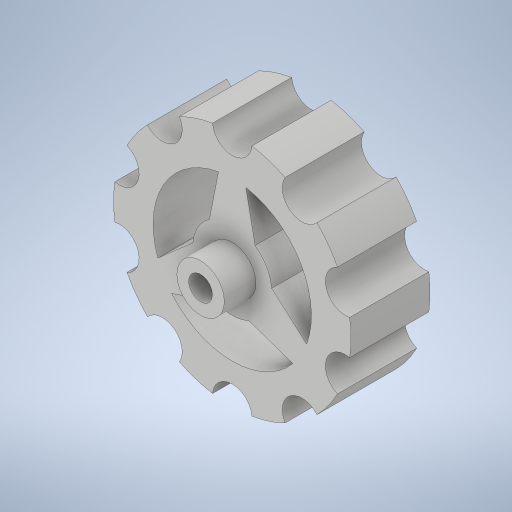
# Autodesk Inventor part: Guntas_Wheel_New
Saved by Autodesk Inventor 2024 (Build 280153000, 153)
## iProperties
Created: 2023-06-29
Part Number: Guntas_Wheel_New
Material: Generic
Document SubType Name: Modeling
Designer: gaura
Density: 1 g/cm^3
Appearance: Default
Author: gaura
Autodesk Inventor part; units mm, degrees
ref_plane "YZ Plane" through (0, 0, 0) normal (1, 0, 0) x (0, 1, 0)
ref_plane "XZ Plane" through (0, 0, 0) normal (0, 1, 0) x (-1, 0, 0)
ref_plane "XY Plane" through (0, 0, 0) normal (0, 0, 1) x (1, 0, 0)
sketch "Sketch1" plane through (0, 0, 0) normal (0, 0, 1) x (1, 0, 0)
  circle A0 centre (0, 0) radius 75
  dimension "d0" = 150
  constraints: 1 centre point, 1 coincident
  measures "d0" diameter of A0
extrude "Extrusion1" add sketch "Sketch1" along normal mid plane 50
sketch "Sketch2" plane through (0, 0, 0) normal (0, 0, 1) x (1, 0, 0)
  circle A0 centre (0, 0) radius 50
  dimension "d3" = 100
  constraints: 1 centre point, 1 coincident
  measures "d3" diameter of A0
extrude "Extrusion2" cut sketch "Sketch2" along normal mid plane 50
sketch "Sketch3" plane through (0, 0, 0) normal (0, 0, 1) x (1, 0, 0)
  circle A0 centre (0, 0) radius 25
  dimension "d6" = 50
  constraints: 1 centre point, 1 coincident
  measures "d6" diameter of A0
extrude "Extrusion3" add sketch "Sketch3" along normal mid plane 50
sketch "Sketch10" plane through (0, 0, 25) normal (0, 0, 1) x (1, 0, 0)
  circle A0 centre (0, 0) radius 75 projected
  circle A1 centre (0, 75) radius 12.5
  circle A2 centre (-44.0839, 60.6763) radius 12.5
  circle A3 centre (-71.3292, 23.1763) radius 12.5
  circle A4 centre (-71.3292, -23.1763) radius 12.5
  circle A5 centre (-44.0839, -60.6763) radius 12.5
  circle A6 centre (0, -75) radius 12.5
  circle A7 centre (44.0839, -60.6763) radius 12.5
  circle A8 centre (71.3292, -23.1763) radius 12.5
  circle A9 centre (71.3292, 23.1763) radius 12.5
  circle A10 centre (44.0839, 60.6763) radius 12.5
  dimension "d46" = 25
  dimension "d49" = 360
  constraints: 10 centre point, 1 vertical alignment, 22 other
  measures "d46" diameter of A1
extrude "Extrusion9" cut sketch "Sketch10" against normal through all contours A9 A0 | A0 A9 | A8 A0 | A0 A8 | A10 A0 | A0 A10 | A7 A0 | A0 A7 | A1 A0 | A0 A1 | A6 A0 | A0 A6 | A2 A0 | A0 A2 | A5 A0 | A0 A5 | A3 A0 | A0 A3 | A4 A0 | A0 A4
sketch "Sketch11" plane through (0, 0, 0) normal (0, 0, 1) x (1, 0, 0)
  circle A0 centre (0, 0) radius 25 construction
  circle A1 centre (0, 0) radius 50 construction
  line L0 (0, 0) -> (50, 0) construction
  line L1 (-8.6824, 49.2404) -> (-14.3982, 20.4375)
  line L2 (8.6824, 49.2404) -> (14.3982, 20.4375)
  line L3 (-38.3022, -32.1394) -> (-10.5003, -22.6879)
  line L4 (-46.9846, -17.101) -> (-24.8985, 2.2504)
  line L5 (46.9846, -17.101) -> (24.8985, 2.2504)
  line L6 (38.3022, -32.1394) -> (10.5003, -22.6879)
  arc A2 (8.6824, 49.2404) -> (-8.6824, 49.2404) centre (0, 0) ccw
  arc A3 (-46.9846, -17.101) -> (-38.3022, -32.1394) centre (0, 0) ccw
  arc A4 (38.3022, -32.1394) -> (50, 0) centre (0, 0) ccw
  arc A5 (10.5003, -22.6879) -> (24.8985, 2.2504) centre (0, 0) ccw
  arc A6 (14.3982, 20.4375) -> (-14.3982, 20.4375) centre (0, 0) ccw
  arc A7 (-24.8985, 2.2504) -> (-10.5003, -22.6879) centre (0, 0) ccw
  dimension "d56" = 360
  constraints: 14 end point, 12 point on circle, 6 centre point, 2 coincident, 1 horizontal, 23 other
extrude "Extrusion10" add sketch "Sketch11" along normal mid plane 50
sketch "Sketch12" plane through (0, 0, 25) normal (0, 0, 1) x (1, 0, 0)
  circle A0 centre (0, 0) radius 15
  dimension "d60" = 30
  constraints: 1 centre point, 1 coincident
  measures "d60" diameter of A0
extrude "Extrusion11" add sketch "Sketch12" along normal blind 20
sketch "Sketch13" plane through (0, 0, 45) normal (0, 0, 1) x (1, 0, 0)
  circle A0 centre (0, 0) radius 7.5
  dimension "d63" = 15
  constraints: 1 centre point, 1 coincident
  measures "d63" diameter of A0
extrude "Extrusion12" cut sketch "Sketch13" against normal blind 20
body "Solid1"
